1.3mm_funnel (Autodesk Fusion 360 design; units mm, degrees)
Autodesk Fusion 360 part; units mm, degrees
sketch "Sketch1" plane through (0, 0, 0) normal (0, 1, 0) x (1, 0, 0)
  line L0 (-9.5, -0.8) -> (-2, -0.8)
  line L1 (-2, -0.8) -> (0, -2.8)
  line L2 (0, -2.8) -> (0, -10)
  line L3 (0, -10) -> (-14, -10)
  line L4 (-14, -10) -> (-14, -8)
  line L5 (-9.5, -0.8) -> (-9.5, -0.6)
  line L6 (-9.5, -0.6) -> (-10, -0.6)
  line L7 (-10, -0.6) -> (-14, -8)
  dimension "d1" = 0.8
  dimension "d2" = 7.5
  dimension "d3" = 2
  dimension "d4" = 2
  dimension "d5" = 10
  dimension "d6" = 2
  dimension "d7" = 14
  dimension "d8" = 0.6
  dimension "d9" = 0.5
  constraint horizontal L0
  constraint perpendicular L0 L2
  constraint perpendicular L2 L3
  constraint perpendicular L3 L4
  constraint coincident origin L2
  constraint perpendicular L0 L5
  constraint perpendicular L5 L6
  measures "d1" distance of origin L0
  measures "d2" distance of L0.start L0.end
  measures "d3" horizontal distance of L0.end L1.end
  measures "d4" vertical distance of L0.end L1.end
  measures "d5" distance of origin L3
  measures "d6" distance of L3 L4.end
  measures "d7" distance of L2.end L3.end
  measures "d8" distance of origin L6
  measures "d9" distance of L5.end L6.end
revolve "Revolve1" add sketch "Sketch1" angle 360 about axis through (1.75, 0, 0) along (1, 0, 0)
sketch "Sketch2" plane through (0, 0, 0) normal (0, 1, 0) x (1, 0, 0)
  line L0 (-12, -2.6074) -> (-1.9501, -2.6074) construction
  line L1 (-1.9501, -2.6074) -> (-1.9501, 2) construction
  line L2 (-1.9501, 2) -> (-12, 2) construction
  line L3 (-12, 2) -> (-12, -2.6074) construction
  dimension "d13" = 2
  text T0 "1.3 mm" font "Arial" height 2 align centre middle in box 10.0499 x 4.6074 at (-12, -2.6074) x (1, 0) y (0, 1) spacing 1
emboss "Emboss1" depth 0.2 profiles "Sketch2" section 1 text T0 onto face at (-4.6667, 0.4985, 9.9876)
fillet "Fillet1" radius 0.5 3 edges at (-14, -3.6162, -9.3233) (-14, -2.8929, -7.4586) (0, -3.6162, -9.3233)
pattern_circular "C-Pattern1" count 3 over 360 about axis through (1.75, 0, 0) along (1, 0, 0) of "Emboss1"
equation "d1 = ( 1.6 / 2 ) * 1 mm"
equation "d8 = 1.2 mm / 2"
